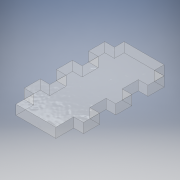
# Autodesk Inventor part: phone_holder_slider_center
Saved by Autodesk Inventor 2019 (Build 230136000, 136)
## iProperties
Created: 2019-02-17
Part Number: phone_holder_slider_center
Material: Acrylic, Clear
Document SubType Name: Modeling
Designer: suchanek
Density: 1.19 g/cm^3
Appearance: Transparent - Clear
Author: suchanek
Autodesk Inventor part; units mm, degrees
ref_plane "YZ Plane" through (0, 0, 0) normal (1, 0, 0) x (0, 1, 0)
ref_plane "XZ Plane" through (0, 0, 0) normal (0, 1, 0) x (-1, 0, 0)
ref_plane "XY Plane" through (0, 0, 0) normal (0, 0, 1) x (1, 0, 0)
sketch "Sketch2" plane through (0, 0, 0) normal (0, 1, 0) x (-1, 0, 0)
  line L0 (18.4, -61.11) -> (12.4, -61.11)
  line L1 (12.4, -61.11) -> (12.4, -51.11)
  line L2 (12.4, -51.11) -> (18.4, -51.11)
  line L3 (18.4, -51.11) -> (18.4, -61.11)
  line L4 (18.4, -41.11) -> (12.4, -41.11)
  line L5 (18.4, -31.11) -> (18.4, -41.11)
  line L6 (12.4, -31.11) -> (18.4, -31.11)
  line L7 (12.4, -41.11) -> (12.4, -31.11)
  line L8 (18.4, -21.11) -> (12.4, -21.11)
  line L9 (18.4, -11.11) -> (18.4, -21.11)
  line L10 (12.4, -11.11) -> (18.4, -11.11)
  line L11 (12.4, -21.11) -> (12.4, -11.11)
  line L12 (12.4, 0) -> (-12.4, 0)
  line L13 (-12.4, 0) -> (-12.4, -67.11)
  line L14 (-12.4, -67.11) -> (12.4, -67.11)
  line L15 (12.4, -67.11) -> (12.4, 0)
  line L16 (0, 0) -> (0, -20.0002)
  line L17 (-18.4, -61.11) -> (-12.4, -61.11)
  line L18 (-12.4, -61.11) -> (-12.4, -51.11)
  line L19 (-12.4, -51.11) -> (-18.4, -51.11)
  line L20 (-18.4, -51.11) -> (-18.4, -61.11)
  line L21 (-18.4, -41.11) -> (-12.4, -41.11)
  line L22 (-18.4, -31.11) -> (-18.4, -41.11)
  line L23 (-12.4, -31.11) -> (-18.4, -31.11)
  line L24 (-12.4, -41.11) -> (-12.4, -31.11)
  line L25 (-18.4, -21.11) -> (-12.4, -21.11)
  line L26 (-18.4, -11.11) -> (-18.4, -21.11)
  line L27 (-12.4, -11.11) -> (-18.4, -11.11)
  line L28 (-12.4, -21.11) -> (-12.4, -11.11)
  point P0 (-12.4, -20.0002)
  point P1 (-18.4, -10)
  dimension "d57" = 6
  dimension "d58" = 10
  dimension "d61" = 20
  dimension "d68" = 24.8
  dimension "d69" = 11.11
  dimension "d70" = 6
  constraints: 58 end point, 12 symmetric about line, 4 parallel, 3 collinear, 2 horizontal, 2 perpendicular, 2 point on line, 2 vertical, 1 midpoint, 15 other
  measures "d57" distance of L1.end L2.end
  measures "d58" distance of L0.end L1.end
  measures "d61" distance of L0.start L4.start
  measures "d68" distance of L13.end L14.end
  measures "d69" distance between parallel lines of L12 L27
  measures "d70" distance between parallel lines of L14 L17
extrude "Extrusion2" add sketch "Sketch2" along normal blind 6
body "Solid2"
